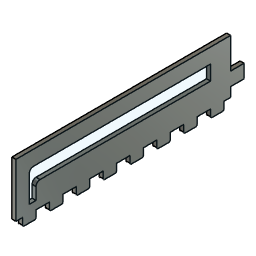
Slingshot Side (Autodesk Fusion 360 design; units mm, degrees)
Autodesk Fusion 360 part; units mm, degrees
sketch "Sketch1" plane through (0, 0, 0) normal (1, 0, 0) x (0, 1, 0)
  line L0 (0, 0) -> (160, 0)
  line L1 (160, 0) -> (160, 40)
  line L2 (160, 40) -> (0, 40)
  line L3 (0, 40) -> (0, 0)
  line L4 (5, 0) -> (5, -5)
  line L5 (6, -6) -> (14, -6)
  line L6 (15, -5) -> (15, 0)
  line L7 (25, 0) -> (35, 0)
  line L8 (35, 0) -> (35, -5)
  line L9 (34, -6) -> (26, -6)
  line L10 (25, -5) -> (25, 0)
  line L11 (45, 0) -> (55, 0)
  line L12 (55, 0) -> (55, -5)
  line L13 (54, -6) -> (46, -6)
  line L14 (45, -5) -> (45, 0)
  line L15 (65, 0) -> (75, 0)
  line L16 (75, 0) -> (75, -5)
  line L17 (74, -6) -> (66, -6)
  line L18 (65, -5) -> (65, 0)
  line L19 (85, 0) -> (95, 0)
  line L20 (95, 0) -> (95, -5)
  line L21 (94, -6) -> (86, -6)
  line L22 (85, -5) -> (85, 0)
  line L23 (105, 0) -> (115, 0)
  line L24 (115, 0) -> (115, -5)
  line L25 (114, -6) -> (106, -6)
  line L26 (105, -5) -> (105, 0)
  line L27 (125, 0) -> (135, 0)
  line L28 (135, 0) -> (135, -5)
  line L29 (134, -6) -> (126, -6)
  line L30 (125, -5) -> (125, 0)
  line L31 (145, 0) -> (155, 0)
  line L32 (155, 0) -> (155, -5)
  line L33 (154, -6) -> (146, -6)
  line L34 (145, -5) -> (145, 0)
  line L35 (15, -2.5) -> (25, -2.5) construction
  line L36 (35, -2.5) -> (45, -2.5) construction
  line L37 (55, -2.5) -> (65, -2.5) construction
  line L38 (75, -2.5) -> (85, -2.5) construction
  line L39 (95, -2.5) -> (105, -2.5) construction
  line L40 (115, -2.4317) -> (125, -2.4308) construction
  line L41 (135, -2.5) -> (145, -2.5054) construction
  line L42 (10, 0) -> (10, 18)
  line L43 (15, 15) -> (15, 0)
  line L44 (10, 6) -> (15, 6)
  line L45 (10, 18) -> (10, 26)
  line L46 (18, 18) -> (145, 18)
  line L47 (145, 18) -> (145, 29)
  line L48 (145, 29) -> (13, 29)
  line L49 (15, 6) -> (160, 6) construction
  line L50 (145, 18) -> (145, 6) construction
  arc A0 (13, 29) -> (10, 26) centre (13, 26) ccw
  arc A1 (18, 18) -> (15, 15) centre (18, 15) ccw
  line L51 (25, 18) -> (25, 0) construction
  line L52 (160, 14.5) -> (160, 9.5) construction
  line L53 (19.9191, 18) -> (19.9191, 6) construction
  line L54 (160, 7) -> (160, 17) construction
  arc A2 (5, -5) -> (6, -6) centre (6, -5) ccw
  arc A3 (14, -6) -> (15, -5) centre (14, -5) ccw
  arc A4 (25, -5) -> (26, -6) centre (26, -5) ccw
  arc A5 (34, -6) -> (35, -5) centre (34, -5) ccw
  arc A6 (45, -5) -> (46, -6) centre (46, -5) ccw
  arc A7 (54, -6) -> (55, -5) centre (54, -5) ccw
  arc A8 (65, -5) -> (66, -6) centre (66, -5) ccw
  arc A9 (74, -6) -> (75, -5) centre (74, -5) ccw
  arc A10 (85, -5) -> (86, -6) centre (86, -5) ccw
  arc A11 (94, -6) -> (95, -5) centre (94, -5) ccw
  arc A12 (105, -5) -> (106, -6) centre (106, -5) ccw
  arc A13 (114, -6) -> (115, -5) centre (114, -5) ccw
  arc A14 (125, -5) -> (126, -6) centre (126, -5) ccw
  arc A15 (134, -6) -> (135, -5) centre (134, -5) ccw
  arc A16 (145, -5) -> (146, -6) centre (146, -5) ccw
  arc A17 (154, -6) -> (155, -5) centre (154, -5) ccw
  line L55 (160, 17) -> (170, 17)
  line L56 (170, 17) -> (170, 7)
  line L57 (170, 7) -> (160, 7)
  line L58 (160, 7) -> (160, 17)
  line L59 (170, 12) -> (19.9191, 12) construction
  point P0 (5, -6)
  point P1 (15, -6)
  point P2 (15, 18)
  point P3 (10, 29)
  dimension "d1" = 160
  dimension "d2" = 40
  dimension "d3" = 10
  dimension "d4" = 6
  dimension "d5" = 5
  dimension "d6" = 10
  dimension "d7" = 5
  dimension "d9" = 18
  dimension "d10" = 5
  dimension "d15" = 11
  dimension "d16" = 130
  dimension "d17" = 12
  dimension "d18" = 3
  dimension "d19" = 3
  dimension "d29" = 1
  dimension "d30" = 1
  dimension "d31" = 1
  dimension "d32" = 1
  dimension "d33" = 1
  dimension "d34" = 1
  dimension "d35" = 1
  dimension "d36" = 1
  dimension "d37" = 1
  dimension "d38" = 1
  dimension "d39" = 1
  dimension "d40" = 1
  dimension "d41" = 1
  dimension "d42" = 1
  dimension "d43" = 1
  dimension "d44" = 1
  dimension "d45" = 10
  dimension "d46" = 10
  constraint horizontal L0
  constraint vertical L1
  constraint horizontal L2
  constraint vertical L3
  constraint coincident L0.start L3.end
  constraint coincident L0 L4.start
  constraint perpendicular L0 L4
  constraint perpendicular L4 L5
  constraint coincident L0 L6.end
  constraint perpendicular L0 L6
  constraint horizontal L7
  constraint vertical L8
  constraint horizontal L9
  constraint vertical L10
  constraint coincident L0 L7.start
  constraint horizontal L11
  constraint vertical L12
  constraint horizontal L13
  constraint vertical L14
  constraint coincident L0 L11.start
  constraint horizontal L15
  constraint vertical L16
  constraint horizontal L17
  constraint vertical L18
  constraint coincident L0 L15.start
  constraint horizontal L19
  constraint vertical L20
  constraint horizontal L21
  constraint vertical L22
  constraint coincident L0 L19.start
  constraint horizontal L23
  constraint vertical L24
  constraint horizontal L25
  constraint vertical L26
  constraint coincident L0 L23.start
  constraint horizontal L27
  constraint vertical L28
  constraint horizontal L29
  constraint vertical L30
  constraint coincident L0 L27.start
  constraint horizontal L31
  constraint vertical L32
  constraint horizontal L33
  constraint vertical L34
  constraint coincident L0 L31.start
  constraint perpendicular L10 L35
  constraint equal L35 L36
  constraint perpendicular L18 L37
  constraint perpendicular L22 L38
  constraint perpendicular L26 L39
  constraint equal L36 L37
  constraint equal L37 L38
  constraint equal L38 L39
  constraint equal L39 L40
  constraint equal L40 L41
  constraint coincident L0 L42.start
  constraint perpendicular L0 L42
  constraint perpendicular L0 L43
  constraint coincident L42 L44.start
  constraint coincident L43 L44.end
  constraint perpendicular L43 L44
  constraint perpendicular L43 L46
  constraint perpendicular L46 L47
  constraint perpendicular L45 L48
  constraint coincident L1 L49.end
  constraint perpendicular L1 L49
  constraint coincident L49 L50.end
  constraint perpendicular L49 L50
  constraint coincident P3 L45
  constraint coincident P3 L48
  constraint tangent L45 A0
  constraint tangent L48 A0
  constraint coincident P2 L43
  constraint coincident P2 L46
  constraint tangent L43 A1
  constraint tangent L46 A1
  constraint coincident L46 L51.start
  constraint equal L42 L51
  constraint perpendicular L46 L51
  constraint perpendicular L47 L48
  constraint vertical L52
  constraint coincident L1 L52.end
  constraint coincident L46 L53.start
  constraint coincident L49 L53.end
  constraint perpendicular L49 L53
  constraint vertical L54
  constraint coincident L52 L54.end
  constraint coincident P0 L4
  constraint coincident P0 L5
  constraint tangent L4 A2
  constraint tangent L5 A2
  constraint coincident L6 L35.start
  constraint coincident P1 L6
  constraint coincident P1 L5
  constraint tangent L6 A3
  constraint tangent L5 A3
  constraint coincident L10 L35.end
  constraint tangent L10 A4
  constraint tangent L9 A4
  constraint coincident L8 L36.start
  constraint tangent L8 A5
  constraint tangent L9 A5
  constraint coincident L14 L36.end
  constraint tangent L14 A6
  constraint tangent L13 A6
  constraint coincident L12 L37.start
  constraint tangent L12 A7
  constraint tangent L13 A7
  constraint coincident L18 L37.end
  constraint tangent L18 A8
  constraint tangent L17 A8
  constraint coincident L16 L38.start
  constraint tangent L16 A9
  constraint tangent L17 A9
  constraint coincident L22 L38.end
  constraint tangent L22 A10
  constraint tangent L21 A10
  constraint coincident L20 L39.start
  constraint tangent L20 A11
  constraint tangent L21 A11
  constraint coincident L26 L39.end
  constraint tangent L26 A12
  constraint tangent L25 A12
  constraint coincident L24 L40.start
  constraint tangent L24 A13
  constraint tangent L25 A13
  constraint coincident L30 L40.end
  constraint tangent L30 A14
  constraint tangent L29 A14
  constraint coincident L28 L41.start
  constraint tangent L28 A15
  constraint tangent L29 A15
  constraint coincident L34 L41.end
  constraint tangent L34 A16
  constraint tangent L33 A16
  constraint tangent L32 A17
  constraint tangent L33 A17
  constraint equal L6 L8
  constraint equal L8 L12
  constraint equal L12 L16
  constraint equal L16 L20
  constraint equal L20 L24
  constraint equal L24 L28
  constraint equal L28 L32
  constraint equal L5 L9
  constraint equal L9 L13
  constraint equal L13 L17
  constraint equal L17 L21
  constraint equal L21 L25
  constraint equal L25 L29
  constraint equal L29 L33
  constraint horizontal L55
  constraint vertical L56
  constraint horizontal L57
  constraint vertical L58
  constraint coincident L54 L55.start
  constraint midpoint L56 L59.start
  constraint midpoint L53 L59.end
  constraint horizontal L59
  measures "d1" distance of L0.start L0.end
  measures "d2" distance of L0.start L2.end
  measures "d3" distance of P0 P1
  measures "d4" distance of L4.start P0
  measures "d5" distance of L0.start L4.start
  measures "d6" distance of L36.start L36.end
  measures "d7" distance of L0.end L32
  measures "d9" distance of L42.start L42.end
  measures "d10" distance of L44.start L44.end
  measures "d15" distance of L42.end P3
  measures "d16" distance of P2 L46.end
  measures "d17" distance of L44 L46
  measures "d18" radius of A0
  measures "d19" radius of A1
  measures "d29" radius of A2
  measures "d30" radius of A3
  measures "d31" radius of A4
  measures "d32" radius of A5
  measures "d33" radius of A6
  measures "d34" radius of A7
  measures "d35" radius of A8
  measures "d36" radius of A9
  measures "d37" radius of A10
  measures "d38" radius of A11
  measures "d39" radius of A12
  measures "d40" radius of A13
  measures "d41" radius of A14
  measures "d42" radius of A15
  measures "d43" radius of A16
  measures "d44" radius of A17
  measures "d45" distance of L54.end L55.end
  measures "d46" distance of L55.end L56.end
extrude "Extrude1" add sketch "Sketch1" along normal blind 3 contours L0 L1 L2 L3 L7 L11 L15 L19 L23 L27 L31 L42 L43 L45 L46 L47 L48 A0 A1 L58 | L0 L4 L5 L6 A2 A3 | L0 L42 L43 L44 | L1 L55 L56 L57 L58 | L0 L7 L8 L9 L10 A4 A5 | L0 L11 L12 L13 L14 A6 A7 | L0 L31 L32 L33 L34 A16 A17 | L0 L15 L16 L17 L18 A8 A9 | L0 L27 L28 L29 L30 A14 A15 | L0 L19 L20 L21 L22 A10 A11 | L0 L23 L24 L25 L26 A12 A13
sketch "Sketch2" plane through (3, 0, 0) normal (1, 0, 0) x (0, 1, 0)
  line L0 (145, 29) -> (145, 18)
  line L1 (145, 18) -> (18, 18)
  arc A0 (18, 18) -> (15, 15) centre (18, 15) ccw
  line L2 (15, 15) -> (15, 6)
  line L3 (15, 6) -> (10, 6)
  line L4 (10, 6) -> (10, 26)
  arc A1 (13, 29) -> (10, 26) centre (13, 26) ccw
  line L5 (13, 29) -> (145, 29)
  line L6 (160, 17) -> (160, 40)
  line L7 (160, 40) -> (0, 40)
  line L8 (0, 40) -> (0, 0)
  line L9 (0, 0) -> (5, 0)
  line L10 (5, 0) -> (5, -5)
  arc A2 (5, -5) -> (6, -6) centre (6, -5) ccw
  line L11 (6, -6) -> (14, -6)
  arc A3 (14, -6) -> (15, -5) centre (14, -5) ccw
  line L12 (15, -5) -> (15, 0)
  line L13 (15, 0) -> (25, 0)
  line L14 (25, 0) -> (25, -5)
  arc A4 (25, -5) -> (26, -6) centre (26, -5) ccw
  line L15 (26, -6) -> (34, -6)
  arc A5 (34, -6) -> (35, -5) centre (34, -5) ccw
  line L16 (35, -5) -> (35, 0)
  line L17 (35, 0) -> (45, 0)
  line L18 (45, 0) -> (45, -5)
  arc A6 (45, -5) -> (46, -6) centre (46, -5) ccw
  line L19 (46, -6) -> (54, -6)
  arc A7 (54, -6) -> (55, -5) centre (54, -5) ccw
  line L20 (55, -5) -> (55, 0)
  line L21 (55, 0) -> (65, 0)
  line L22 (65, 0) -> (65, -5)
  arc A8 (65, -5) -> (66, -6) centre (66, -5) ccw
  line L23 (66, -6) -> (74, -6)
  arc A9 (74, -6) -> (75, -5) centre (74, -5) ccw
  line L24 (75, -5) -> (75, 0)
  line L25 (75, 0) -> (85, 0)
  line L26 (85, 0) -> (85, -5)
  arc A10 (85, -5) -> (86, -6) centre (86, -5) ccw
  line L27 (86, -6) -> (94, -6)
  arc A11 (94, -6) -> (95, -5) centre (94, -5) ccw
  line L28 (95, -5) -> (95, 0)
  line L29 (95, 0) -> (105, 0)
  line L30 (105, 0) -> (105, -5)
  arc A12 (105, -5) -> (106, -6) centre (106, -5) ccw
  line L31 (106, -6) -> (114, -6)
  arc A13 (114, -6) -> (115, -5) centre (114, -5) ccw
  line L32 (115, -5) -> (115, 0)
  line L33 (115, 0) -> (125, 0)
  line L34 (125, 0) -> (125, -5)
  arc A14 (125, -5) -> (126, -6) centre (126, -5) ccw
  line L35 (126, -6) -> (134, -6)
  arc A15 (134, -6) -> (135, -5) centre (134, -5) ccw
  line L36 (135, -5) -> (135, 0)
  line L37 (135, 0) -> (145, 0)
  line L38 (145, 0) -> (145, -5)
  arc A16 (145, -5) -> (146, -6) centre (146, -5) ccw
  line L39 (146, -6) -> (154, -6)
  arc A17 (154, -6) -> (155, -5) centre (154, -5) ccw
  line L40 (155, -5) -> (155, 0)
  line L41 (155, 0) -> (160, 0)
  line L42 (160, 0) -> (160, 7)
  line L43 (160, 7) -> (170, 7)
  line L44 (170, 7) -> (170, 17)
  line L45 (170, 17) -> (160, 17)
